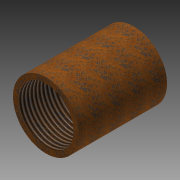
# Autodesk Inventor part: Pipe Fitting
Saved by Autodesk Inventor 2013 SP2 (Build 170200200, 200)
## iProperties
Created: 2014-06-02
Part Number: Pipe Fitting
Material: Steel
Document SubType Name: Modeling
Designer: jmw3
Mass: 138.92 g
Surface Area: 118.443 cm^2
Volume: 17.6968 cm^3
Density: 7.85 g/cm^3
Author: jmw3
Autodesk Inventor part; units mm, degrees
ref_plane "YZ Plane" through (0, 0, 0) normal (1, 0, 0) x (0, 1, 0)
ref_plane "XZ Plane" through (0, 0, 0) normal (0, 1, 0) x (-1, 0, 0)
ref_plane "XY Plane" through (0, 0, 0) normal (0, 0, 1) x (1, 0, 0)
sketch "Sketch1" plane through (0, 0, 0) normal (0, 0, 1) x (1, 0, 0)
  line L0 (0, -26.67) -> (0, 26.67) projected
  line L1 (-26.67, 0) -> (26.67, 0) projected
  circle A0 centre (0, 0) radius 19.05
  circle A1 centre (0, 0) radius 15.875
  dimension "d0" = 38.1
  dimension "d1" = 31.75
  constraints: 2 centre point, 2 coincident
  measures "d0" diameter of A0
  measures "d1" diameter of A1
extrude "Extrusion1" add sketch "Sketch1" along normal blind 25.4 and the other way blind 25.4 contours A0 L1 A1 L0 | L0 A1 L1 A0 | A0 L0 A1 L1 | L1 A1 L0 A0
thread "Thread1" size "1 1/4" designation "1 1/4 - 11.5 NPT" standard "NPT" length 25.6286
thread "Thread2" size "1 1/4" designation "1 1/4 - 11.5 NPT" standard "NPT" length 25.6286
body "Solid1"
